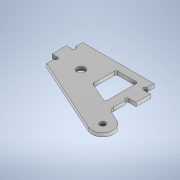
# Autodesk Inventor part: Leg_joint_pitch_frame
Saved by Autodesk Inventor 2020 (Build 240168000, 168)
## iProperties
Created: 2021-09-05
Part Number: Leg_joint_pitch_frame
Material: アルミニウム 2014-T4
Document SubType Name: Modeling
Designer: Masato Kubotera
Density: 2.8 g/cm^3
Appearance: 滑らか - 淡い灰色
Mass: 6.13105 g
Surface Area: 26.9426 cm^2
Volume: 2.18966 cm^3
Description: A2017 T2
Author: Masato Kubotera
Title: 付け根_メインフレーム_1
Autodesk Inventor part; units mm, degrees
ref_plane "YZ Plane" through (0, 0, 0) normal (1, 0, 0) x (0, 1, 0)
ref_plane "XZ Plane" through (0, 0, 0) normal (0, 1, 0) x (-1, 0, 0)
ref_plane "XY Plane" through (0, 0, 0) normal (0, 0, 1) x (1, 0, 0)
sketch "スケッチ1" plane through (0, 0, 0) normal (0, 0, 1) x (1, 0, 0)
  line L0 (-19.75, 25.75) -> (19.75, 25.75) construction
  line L1 (19.75, 25.75) -> (19.75, -25.75) construction
  line L2 (19.75, -25.75) -> (-19.75, -25.75) construction
  line L3 (-19.75, -25.75) -> (-19.75, 25.75) construction
  line L4 (-19.75, 25.75) -> (19.75, -25.75) construction
  line L5 (19.75, 25.75) -> (-19.75, -25.75) construction
  circle A0 centre (24.75, -24.25) radius 1.55
  circle A1 centre (-7.25, -4.25) radius 2.25
  line L6 (0, 25.75) -> (0, -25.75) construction
  line L7 (-19.75, 3.25) -> (-22.75, 3.25)
  line L8 (-22.75, 3.25) -> (-22.75, -4.75)
  arc A2 (-19.75, 3.25) -> (-19.75, 5.35) centre (-19.75, 4.3) ccw
  line L9 (-22.75, -0.75) -> (-19.75, -0.75) construction
  line L10 (-19.75, -4.75) -> (-22.75, -4.75)
  arc A3 (-19.75, -6.85) -> (-19.75, -4.75) centre (-19.75, -5.8) ccw
  line L11 (-19.75, 5.35) -> (-19.75, 9.25)
  line L12 (-19.75, 9.25) -> (19.75, 9.25)
  arc A4 (19.75, 5.35) -> (19.75, 3.25) centre (19.75, 4.3) ccw
  arc A5 (19.75, -4.75) -> (19.75, -6.85) centre (19.75, -5.8) ccw
  line L13 (19.75, 5.35) -> (19.75, 9.25)
  arc A6 (22.2819, -29.7189) -> (27.2181, -18.7811) centre (24.75, -24.25) ccw
  line L14 (-19.75, -6.85) -> (-19.75, -10.75)
  line L15 (-19.75, -10.75) -> (22.2819, -29.7189)
  line L16 (19.75, -6.85) -> (19.75, -15.4108)
  line L17 (19.75, -15.4108) -> (27.2181, -18.7811)
  circle A7 centre (-7.25, -4.25) radius 6 construction
  circle A8 centre (24.75, -24.25) radius 6 construction
  line L18 (2.75, 5.25) -> (14.75, 5.25)
  line L19 (14.75, 5.25) -> (14.75, -13.1543)
  line L20 (14.75, -13.1543) -> (2.75, -7.7388)
  line L21 (2.75, -7.7388) -> (2.75, 5.25)
  line L22 (19.75, 3.25) -> (23.75, 3.25)
  line L23 (23.75, 3.25) -> (23.75, -4.75)
  line L24 (23.75, -4.75) -> (19.75, -4.75)
  point P0 (0, 0)
  dimension "d0" = 39.5
  dimension "d1" = 51.5
  dimension "d2" = 3.1
  dimension "d3" = 4.5
  dimension "d4" = 32
  dimension "d5" = 20
  dimension "d6" = 3
  dimension "d7" = 1.05
  dimension "d8" = 8
  dimension "d9" = 26.5
  dimension "d11" = 30
  dimension "d12" = 12.5
  dimension "d13" = 6
  dimension "d14" = 12
  dimension "d19" = 12
  dimension "d20" = 12
  dimension "d21" = 4
  dimension "d22" = 5
  dimension "d24" = 4
  dimension "d26" = 4
  constraints: 50 end point, 10 point on circle, 10 symmetric about line, 9 centre point, 7 perpendicular, 7 point on line, 5 midpoint, 5 parallel, 4 horizontal, 3 coincident, 2 tangent, 1 collinear, 3 other
  measures "d0" distance of L1.end L2.end
  measures "d1" distance of L0.end L1.end
  measures "d2" diameter of A0
  measures "d3" diameter of A1
  measures "d4" horizontal distance of A0.centre A1.centre
  measures "d5" vertical distance of A0.centre A1.centre
  measures "d6" distance of L7.start L7.end
  measures "d7" radius of A2
  measures "d8" distance of L7.end L8.end
  measures "d9" vertical distance of L0.start L9.start
  measures "d11" vertical distance of L0.start A1.centre
  measures "d12" horizontal distance of A1.centre L0.start
  measures "d13" vertical distance of L7.end L11.end
  measures "d14" diameter of A6
  measures "d19" diameter of A7
  measures "d20" diameter of A8
  measures "d21" distance between parallel lines of L18 L12
  measures "d22" distance between parallel lines of L1 L19
  measures "d24" distance edge to line of A7 L21
  measures "d26" distance between parallel lines of L1 L23
extrude "押し出し1" add sketch "スケッチ1" along normal blind 2
fillet "フィレット1" radius 3.5 1 edges at (19.75, -15.4108, 1)
fillet "フィレット2" radius 1 4 edges at (2.75, 5.25, 1) (14.75, 5.25, 1) (2.75, -7.7388, 1) (14.75, -13.1543, 1)
equation "\"d24\" = d21"
